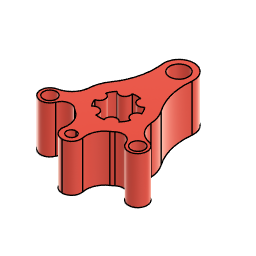
chan edm v1 (Autodesk Fusion 360 design; units mm, degrees)
Autodesk Fusion 360 part; units mm, degrees
sketch "Sketch1" plane through (0, 0, 0) normal (0, 0, 1) x (1, 0, 0)
  circle A0 centre (0, 65) radius 10
  circle A1 centre (-47, -26) radius 7
  arc A2 (-27.0298, 18.9312) -> (-15.8903, 63.1292) centre (-79.4513, 55.6462) ccw
  circle A3 centre (-0.1967, -50) radius 5
  arc A4 (-48.9633, -16.1946) -> (-32.9314, 2.127) centre (-52.8898, 3.4162) ccw
  arc A5 (-9.9929, -47.9913) -> (-18.421, -27.38) centre (-29.5853, -43.974) ccw
  arc A6 (-21.5665, -24.9777) -> (-37.5509, -29.2733) centre (-28.1018, -32.5467) ccw
  arc A7 (-19.1, -5.9321) -> (-19.1, 5.9321) centre (-20, 0) ccw
  arc A8 (-19.1, -5.9321) -> (-19.1, 5.9321) centre (-20, 0) ccw
  arc A9 (-19.1, -5.9321) -> (-19.1, 5.9321) centre (-20, 0) ccw
  arc A10 (-19.1, -5.9321) -> (-19.1, 5.9321) centre (-20, 0) ccw
  arc A11 (-4.4126, -19.5071) -> (-14.6874, -13.575) centre (-10, -17.3205) ccw
  arc A12 (14.6874, -13.575) -> (4.4126, -19.5071) centre (10, -17.3205) ccw
  arc A13 (-19.1, -5.9321) -> (-19.1, 5.9321) centre (-20, 0) ccw
  arc A14 (-19.1, -5.9321) -> (-14.6874, -13.575) centre (0, 0) ccw
  arc A15 (-14.6874, 13.575) -> (-4.4126, 19.5071) centre (-10, 17.3205) ccw
  arc A16 (-14.6874, 13.575) -> (-19.1, 5.9321) centre (0, 0) ccw
  arc A17 (4.4126, 19.5071) -> (14.6874, 13.575) centre (10, 17.3205) ccw
  arc A18 (4.4126, 19.5071) -> (-4.4126, 19.5071) centre (0, 0) ccw
  arc A19 (19.1, 5.9321) -> (19.1, -5.9321) centre (20, 0) ccw
  arc A20 (19.1, 5.9321) -> (14.6874, 13.575) centre (0, 0) ccw
  arc A21 (-4.4126, -19.5071) -> (4.4126, -19.5071) centre (0, 0) ccw
  arc A22 (14.6874, -13.575) -> (19.1, -5.9321) centre (0, 0) ccw
  arc A23 (-19.1, -5.9321) -> (-19.1, 5.9321) centre (-20, 0) ccw
  circle A24 centre (0, 65) radius 10
  arc A25 (15.8903, 63.1292) -> (27.0298, 18.9312) centre (79.4513, 55.6462) ccw
  arc A26 (32.9314, 2.127) -> (48.9633, -16.1946) centre (52.8898, 3.4162) ccw
  circle A27 centre (47, -26) radius 7
  arc A28 (37.5509, -29.2733) -> (21.5665, -24.9777) centre (28.1018, -32.5467) ccw
  arc A29 (18.421, -27.38) -> (9.9929, -47.9913) centre (29.5853, -43.974) ccw
  arc A30 (14.6874, -13.575) -> (19.1, -5.9321) centre (0, 0) ccw
  arc A31 (19.1, 5.9321) -> (19.1, -5.9321) centre (20, 0) ccw
  arc A32 (19.1, 5.9321) -> (14.6874, 13.575) centre (0, 0) ccw
  arc A33 (4.4126, 19.5071) -> (14.6874, 13.575) centre (10, 17.3205) ccw
  arc A34 (4.4126, 19.5071) -> (-4.4126, 19.5071) centre (0, 0) ccw
  arc A35 (-4.4126, -19.5071) -> (4.4126, -19.5071) centre (0, 0) ccw
  arc A36 (14.6874, -13.575) -> (4.4126, -19.5071) centre (10, -17.3205) ccw
  circle A37 centre (0.1967, -50) radius 5
  arc A38 (-4.4126, -19.5071) -> (-14.6874, -13.575) centre (-10, -17.3205) ccw
  arc A39 (-19.1, -5.9321) -> (-14.6874, -13.575) centre (0, 0) ccw
  arc A40 (-19.1, -5.9321) -> (-19.1, 5.9321) centre (-20, 0) ccw
  arc A41 (-14.6874, 13.575) -> (-4.4126, 19.5071) centre (-10, 17.3205) ccw
  arc A42 (-14.6874, 13.575) -> (-19.1, 5.9321) centre (0, 0) ccw
  arc A43 (-27.0298, 18.9312) -> (-32.9314, 2.127) centre (0, 0) ccw
  arc A44 (-27.0298, 18.9312) -> (-32.9314, 2.127) centre (0, 0) ccw
  arc A45 (-21.5665, -24.9777) -> (-18.421, -27.38) centre (0, 0) ccw
  arc A46 (-21.5665, -24.9777) -> (-18.421, -27.38) centre (0, 0) ccw
  arc A47 (18.421, -27.38) -> (21.5665, -24.9777) centre (0, 0) ccw
  arc A48 (32.9314, 2.127) -> (27.0298, 18.9312) centre (0, 0) ccw
  arc A49 (18.421, -27.38) -> (21.5665, -24.9777) centre (0, 0) ccw
  arc A50 (32.9314, 2.127) -> (27.0298, 18.9312) centre (0, 0) ccw
  arc A51 (-9.9929, -47.9913) -> (0, -59.9981) centre (-0.1967, -50) ccw
  arc A52 (0, -59.9981) -> (9.9929, -47.9913) centre (0.1967, -50) ccw
  arc A53 (-48.9633, -16.1946) -> (-37.5509, -29.2733) centre (-47, -26) ccw
  arc A54 (37.5509, -29.2733) -> (48.9633, -16.1946) centre (47, -26) ccw
  arc A55 (15.8903, 63.1292) -> (-15.8903, 63.1292) centre (0, 65) ccw
  arc A56 (15.8903, 63.1292) -> (-15.8903, 63.1292) centre (0, 65) ccw
  dimension "d1" = 20
  dimension "d2" = 65
  dimension "d3" = 32
  dimension "d4" = 40
  dimension "d5" = 66
  dimension "d6" = 128
  dimension "d7" = 14
  dimension "d8" = 47
  dimension "d9" = 26
  dimension "d10" = 20
  dimension "d11" = 40
  dimension "d12" = 10
  dimension "d13" = 50
  dimension "d14" = 20
  dimension "d15" = 40
  dimension "d16" = 20
  dimension "d17" = 12
  dimension "d21" = 360
  constraint concentric A0 A55
  constraint coincident A14.centre A16.centre
  constraint concentric A21 A44
  constraint tangent A2 A55
  constraint tangent A2 A44
  constraint concentric A1 A53
  constraint tangent A4 A44
  constraint tangent A4 A53
  constraint concentric A3 A51
  constraint tangent A5 A51
  constraint tangent A5 A44
  constraint coincident A5.end A44
  constraint tangent A6 A44
  constraint tangent A6 A53
  constraint coincident A6.start A44
  constraint coincident A7.centre A21
  constraint coincident A7.start A21
  constraint coincident A12.start A21
  constraint concentric A14 A21
  constraint coincident A15.start A21
  constraint concentric A16 A21
  constraint coincident A17.start A21
  constraint concentric A18 A21
  constraint coincident A19.start A21
  constraint concentric A20 A21
  constraint concentric A21 A22
  constraint concentric A43 A45
  constraint concentric A44 A46
  constraint concentric A45 A49
  constraint concentric A46 A47
  constraint concentric A47 A48
  constraint concentric A49 A50
  measures "d1" diameter of A0
  measures "d2" distance of A14.centre A0.centre
  measures "d3" diameter of A55
  measures "d4" diameter of A21
  measures "d5" diameter of A44
  measures "d6" diameter of A2
  measures "d7" diameter of A1
  measures "d8" horizontal distance of A14.centre A1.centre
  measures "d9" vertical distance of A14.centre A1.centre
  measures "d10" diameter of A53
  measures "d11" diameter of A4
  measures "d12" diameter of A3
  measures "d13" vertical distance of A14.centre A3.centre
  measures "d14" diameter of A51
  measures "d15" diameter of A5
  measures "d16" diameter of A6
  measures "d17" diameter of A7
sketch "Sketch2" plane through (0, 0, 0) normal (0, 0, 1) x (1, 0, 0)
sketch "Sketch3" plane through (0, 0, 0) normal (0, 0, 1) x (1, 0, 0)
extrude "Extrude1" add sketch "Sketch1" along normal blind 50
